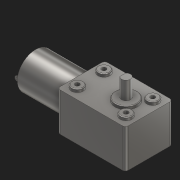
# Autodesk Inventor part: uxcell 12V 6RPM 6mm Worm Gear Motor
Saved by Autodesk Inventor 2017 SP1 (Build 210196100, 196)
## iProperties
Created: 2017-11-07
Part Number: uxcell 12V 6RPM 6mm Worm Gear Motor
Material: Stainless Steel
Document SubType Name: Modeling
Designer: Zach
Density: 8 g/cm^3
Appearance: Semi-Polished
Author: Zach
Autodesk Inventor part; units mm, degrees
ref_plane "YZ Plane" through (0, 0, 0) normal (1, 0, 0) x (0, 1, 0)
ref_plane "XZ Plane" through (0, 0, 0) normal (0, 1, 0) x (-1, 0, 0)
ref_plane "XY Plane" through (0, 0, 0) normal (0, 0, 1) x (1, 0, 0)
sketch "Sketch1" plane through (0, 0, 0) normal (0, 0, 1) x (1, 0, 0)
  line L0 (0, 0) -> (46, 0)
  line L1 (46, 0) -> (46, 32)
  line L2 (46, 32) -> (0, 32)
  line L3 (0, 32) -> (0, 0)
  line L4 (6.5, 25) -> (39.5, 25) construction
  line L5 (39.5, 25) -> (39.5, 7) construction
  line L6 (39.5, 7) -> (6.5, 7) construction
  line L7 (6.5, 7) -> (6.5, 25) construction
  circle A0 centre (39.5, 25) radius 1.5
  circle A1 centre (39.5, 7) radius 1.5
  circle A2 centre (6.5, 25) radius 1.5
  circle A3 centre (6.5, 7) radius 1.5
  point P0 (39.5, 16)
  point P1 (0, 16)
  point P2 (23, 25)
  point P3 (23, 32)
  dimension "d0" = 46
  dimension "d1" = 32
  dimension "d2" = 33
  dimension "d3" = 18
  dimension "d4" = 3
  dimension "d5" = 3
  dimension "d6" = 3
  dimension "d7" = 3
  constraints: 16 end point, 4 centre point, 4 coincident, 4 midpoint, 4 parallel, 2 horizontal, 2 perpendicular, 1 horizontal alignment, 1 vertical alignment
  measures "d0" distance of L2.end L1.end
  measures "d1" distance of L1.end L0.end
  measures "d2" distance of L5.end L6.end
  measures "d3" distance of L4.end L5.end
  measures "d4" diameter of A0
  measures "d5" diameter of A1
  measures "d6" diameter of A2
  measures "d7" diameter of A3
extrude "Extrusion1" add sketch "Sketch1" along normal blind 26
sketch "Sketch2" plane through (0, 0, 26) normal (0, 0, 1) x (1, 0, 0)
  circle A0 centre (30.5, 16) radius 3
  line L0 (46, 0) -> (46, 32) projected
  circle A1 centre (39.5, 25) radius 1.5 projected
  point P0 (0, 0)
  point P1 (46, 16)
  dimension "d10" = 6
  dimension "d12" = 9
  constraints: 1 centre point, 1 horizontal alignment, 1 midpoint
  measures "d10" diameter of A0
  measures "d12" horizontal distance of A1.centre A0.centre
extrude "Extrusion2" add sketch "Sketch2" along normal blind 14 contours A0
sketch "Sketch3" plane through (0, 0, 26) normal (0, 0, 1) x (1, 0, 0)
  circle A0 centre (30.5, 16) radius 3 projected
  circle A1 centre (30.5, 16) radius 7.5
  point P0 (0, 0)
  dimension "d15" = 15
  constraints: 1 centre point, 1 coincident
  measures "d15" diameter of A1
extrude "Extrusion3" add sketch "Sketch3" along normal blind 2
fillet "Fillet1" radius 2 4 edges at (46, 32, 13) (46, 0, 13) (0, 32, 13) (0, 0, 13)
sketch "Sketch4" plane through (0, 2, 0) normal (-1, 0, 0) x (0, 0, 1)
  circle A0 centre (13, 14) radius 12.2
  line L0 (0, 28) -> (0, 0) projected
  line L1 (26, 30) -> (0, 30) projected
  point P0 (0, -2)
  point P1 (0, 14)
  point P2 (13, 30)
  dimension "d19" = 24.4
  constraints: 2 midpoint, 1 centre point, 1 horizontal alignment, 1 vertical alignment
  measures "d19" diameter of A0
extrude "Extrusion4" add sketch "Sketch4" along normal blind 30.8
sketch "Sketch5" plane through (30.5, 16, 40) normal (0, 0, 1) x (1, 0, 0)
  circle A0 centre (0, 0) radius 3 construction
  line L0 (-2.2, 2.0396) -> (-2.2, -2.0396)
  arc A1 (-2.2, 2.0396) -> (-2.2, -2.0396) centre (0, 0) ccw
  point P0 (-30.5, -16)
  dimension "d22" = 2.2
  constraints: 4 point on circle, 2 end point, 1 centre point, 1 concentric, 1 vertical
  measures "d22" distance from line of A0.centre L0
extrude "Extrusion5" cut sketch "Sketch5" against normal blind 8
sketch "Sketch6" plane through (0, 0, 26) normal (0, 0, 1) x (1, 0, 0)
  circle A0 centre (39.5, 25) radius 1.5 projected
  circle A1 centre (39.5, 7) radius 1.5 projected
  circle A2 centre (6.5, 7) radius 1.5 projected
  circle A3 centre (6.5, 25) radius 1.5 projected
  circle A4 centre (6.5, 25) radius 4
  circle A5 centre (6.5, 7) radius 4
  circle A6 centre (39.5, 7) radius 4
  circle A7 centre (39.5, 25) radius 4
  point P0 (0, 0)
  dimension "d25" = 8
  dimension "d26" = 8
  dimension "d27" = 8
  dimension "d28" = 8
  constraints: 4 centre point, 4 coincident
  measures "d25" diameter of A4
  measures "d26" diameter of A5
  measures "d27" diameter of A6
  measures "d28" diameter of A7
extrude "Extrusion6" add sketch "Sketch6" along normal blind 2
sketch "Sketch8" plane through (0, 0, 0) normal (0, 0, -1) x (-1, 0, 0)
  circle A0 centre (-6.5, 7) radius 1.5 projected
  circle A1 centre (-6.5, 25) radius 1.5 projected
  circle A2 centre (-39.5, 7) radius 1.5 projected
  circle A3 centre (-39.5, 25) radius 1.5 projected
  arc A4 (-2, 0) -> (0, 2) centre (-2, 2) ccw construction
  line L0 (0, 30) -> (0, 2) construction
  arc A5 (0, 30) -> (-2, 32) centre (-2, 30) ccw construction
  line L1 (-44, 32) -> (-2, 32) construction
  arc A6 (-44, 32) -> (-46, 30) centre (-44, 30) ccw construction
  line L2 (-46, 2) -> (-46, 30) construction
  arc A7 (-46, 2) -> (-44, 0) centre (-44, 2) ccw construction
  line L3 (-2, 0) -> (-44, 0) construction
  point P0 (0, 0)
extrude "Extrusion7" add sketch "Sketch8" against normal blind 14
fillet "Fillet2" radius 0.5 5 edges at (35.5, 25, 28) (35.5, 7, 28) (2.5, 7, 28) (2.5, 25, 28) (23, 16, 28)
sketch "Sketch9" plane through (-30.8, 16, 13) normal (-1, 0, 0) x (0, 0, 1)
  line L0 (-1.5, 11) -> (1.5, 11)
  line L1 (1.5, 11) -> (1.5, 10.5)
  line L2 (1.5, 10.5) -> (-1.5, 10.5)
  line L3 (-1.5, 10.5) -> (-1.5, 11)
  line L4 (-1.5, -10.5) -> (1.5, -10.5)
  line L5 (1.5, -10.5) -> (1.5, -11)
  line L6 (1.5, -11) -> (-1.5, -11)
  line L7 (-1.5, -11) -> (-1.5, -10.5)
  circle A0 centre (0, 0) radius 12.2 construction
  point P0 (-13, -16)
  point P1 (0, 10.5)
  dimension "d34" = 3
  dimension "d35" = 0.5
  dimension "d36" = 3
  dimension "d37" = 0.5
  dimension "d38" = 10.5
  dimension "d39" = 10.5
  constraints: 16 end point, 4 parallel, 2 horizontal, 2 perpendicular, 1 midpoint, 1 point on line, 1 vertical alignment
  measures "d34" distance of L1.end L2.end
  measures "d35" distance of L0.end L1.end
  measures "d36" distance of L5.end L6.end
  measures "d37" distance of L4.end L5.end
  measures "d38" distance of A0.centre point (0, 10.5)
  measures "d39" distance from line of L4 A0.centre
extrude "Extrusion8" add sketch "Sketch9" along normal blind 3
sketch "Sketch10" plane through (-30.8, 26.5, 11.5) normal (0, -1, 0) x (1, 0, 0)
  circle A0 centre (-1.5, 1.5) radius 1.5 construction
  line L0 (0, 3) -> (-3, 3) construction
  line L1 (0, 0) -> (-3, 0) construction
  line L2 (-3, 3) -> (-3, 0) construction
  circle A1 centre (-1.5, 1.5) radius 0.5
  line L3 (-1.5, 0) -> (-3, 0)
  line L4 (-3, 0) -> (-3, 1.5)
  line L5 (-3, 1.5) -> (-3, 3)
  line L6 (-1.5, 3) -> (-3, 3)
  arc A2 (-1.5, 3) -> (-3, 1.5) centre (-1.5, 1.5) ccw
  arc A3 (-3, 1.5) -> (-1.5, 0) centre (-1.5, 1.5) ccw
  point P0 (30.8, -11.5)
  dimension "d43" = 1
  constraints: 8 end point, 8 tangent, 4 centre point, 4 point on circle, 3 collinear, 3 midpoint, 1 coincident, 1 concentric
  measures "d43" diameter of A1
extrude "Extrusion9" cut sketch "Sketch10" along normal through all both and the other way through all
sketch "Sketch11" plane through (-30.8, 16, 13) normal (-1, 0, 0) x (0, 0, 1)
  circle A0 centre (0, 0) radius 3
  circle A1 centre (0, 0) radius 12.2 construction
  point P0 (-13, -16)
  dimension "d46" = 6
  constraints: 1 centre point, 1 coincident
  measures "d46" diameter of A0
extrude "Extrusion10" add sketch "Sketch11" along normal blind 1
fillet "Fillet4" radius 0.5 1 edges at (-31.8, 16, 10)
body "Solid1"
